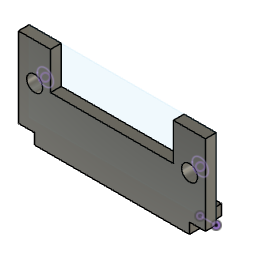
range finder mount update (Autodesk Fusion 360 design; units mm, degrees)
Autodesk Fusion 360 part; units mm, degrees
note: some values were not read from the file. Chosen so that the rebuilt part matches the saved one: which face or edge a step refers to.
sketch "Sketch1" plane through (0, 0, 0) normal (0, 0, 1) x (1, 0, 0)
  circle A0 centre (-75, 25.7988) radius 1.5
  circle A1 centre (-50, 25.7988) radius 1.5
  line L0 (-77, 28) -> (-48, 28)
  line L1 (-48, 28) -> (-48, 22)
  line L2 (-48, 22) -> (-77, 22)
  line L3 (-77, 22) -> (-77, 28)
  dimension "d1" = 25
  dimension "d2" = 3
  dimension "d3" = 3
  constraint horizontal L0
  constraint vertical L1
  constraint horizontal L2
  constraint vertical L3
  measures "d1" distance of A0.centre A1.centre
  measures "d2" diameter of A0
  measures "d3" diameter of A1
extrude "Extrude1" add sketch "Sketch1" along normal blind 2
sketch "Sketch2" plane through (0, 0, 2) normal (0, 0, 1) x (-1, 0, 0)
  circle A0 centre (75, -25.7988) radius 1.5
  circle A1 centre (50, -25.7988) radius 1.5
  line L0 (77, -22) -> (48, -22)
  line L1 (48, -22) -> (48, -28)
  line L2 (48, -28) -> (77, -28)
  line L3 (77, -28) -> (77, -22)
  line L4 (48, -22) -> (77, -22)
  line L5 (77, -22) -> (77, -23)
  line L6 (77, -23) -> (48, -23)
  line L7 (48, -23) -> (48, -22)
  constraint horizontal L4
  constraint vertical L5
  constraint horizontal L6
  constraint vertical L7
  constraint coincident L3 L5.end
  constraint coincident L0.end L1.start
sketch "Sketch3" plane through (0, 23, 0) normal (0, 1, 0) x (-1, 0, 0)
  line L0 (48, 2) -> (77, 2)
  line L1 (77, 17) -> (48, 17)
  circle A0 through (49.472, 10, 1) (47.222, 11.299, 1) (47.222, 8.701, 1)
  circle A1 through (78.472, 10, 1) (76.222, 11.299, 1) (76.222, 8.701, 1)
  line L2 (45, 17, 1) -> (80, 17, 1)
  line L3 (80, 17, 1) -> (80, 2, 1)
  line L4 (80, 2, 1) -> (45, 2, 1)
  line L5 (45, 2, 1) -> (45, 17, 1)
  dimension "d8" = 29
  dimension "d9" = 3
  dimension "d10" = 3
sketch "Sketch3 (curves 1 mm off its plane)" plane through (0, 24, 0) normal (0, 1, 0) x (-1, 0, 0)
  circle A0 centre (47.972, 10) radius 1.5
  circle A1 centre (76.972, 10) radius 1.5
  line L0 (45, 17) -> (80, 17)
  line L1 (80, 17) -> (80, 2)
  line L2 (80, 2) -> (45, 2)
  line L3 (45, 2) -> (45, 17)
extrude "Extrude3" add sketch "Sketch3 (curves 1 mm off its plane)" against normal blind 2
sketch "Sketch4" plane through (0, 24, 0) normal (0, 1, 0) x (-1, 0, 0)
  line L0 (80, 17) -> (45, 17)
  line L1 (45, 17) -> (45, 2)
  line L2 (77, 2) -> (80, 2)
  line L3 (48, 2) -> (77, 2)
  line L4 (80, 2) -> (80, 17)
  circle A0 centre (47.972, 10) radius 1.5
  circle A1 centre (76.972, 10) radius 1.5
  line L5 (45, 2) -> (48, 2)
sketch "Sketch5" plane through (0, 24, 0) normal (0, 1, 0) x (-1, 0, 0)
sketch "Sketch6" plane through (0, 24, 0) normal (0, 1, 0) x (-1, 0, 0)
  line L0 (51, 17, 2) -> (74, 17, 2)
  line L1 (74, 17, 2) -> (74, 10, 2)
  line L2 (74, 10, 2) -> (51, 10, 2)
  line L3 (51, 10, 2) -> (51, 17, 2)
sketch "Sketch6 (curves 2 mm off its plane)" plane through (0, 26, 0) normal (0, 1, 0) x (-1, 0, 0)
  line L0 (51, 17) -> (74, 17)
  line L1 (74, 17) -> (74, 10)
  line L2 (74, 10) -> (51, 10)
  line L3 (51, 10) -> (51, 17)
extrude "Extrude4" cut sketch "Sketch6 (curves 2 mm off its plane)" against normal blind 4
